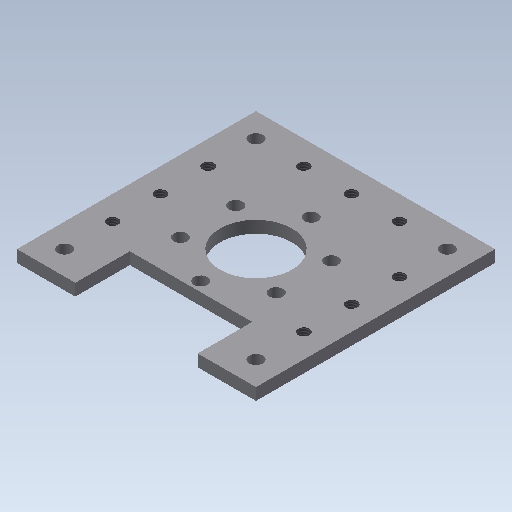
# Autodesk Inventor part: basenueva(5x5)
Saved by Autodesk Inventor 2020 (Build 240168000, 168)
## iProperties
Created: 2016-08-12
Part Number: basenueva(5x5)
Material: Genérico
Document SubType Name: Modeling
Designer: Diego Martinez
Density: 1 g/cm^3
Appearance: Por defecto
Author: Diego Martinez
Autodesk Inventor part; units mm, degrees
ref_plane "YZ Plane" through (0, 0, 0) normal (1, 0, 0) x (0, 1, 0)
ref_plane "XZ Plane" through (0, 0, 0) normal (0, 1, 0) x (-1, 0, 0)
ref_plane "XY Plane" through (0, 0, 0) normal (0, 0, 1) x (1, 0, 0)
sketch "Sketch3" plane through (0, 0, 0) normal (0, 1, 0) x (-1, 0, 0)
  circle A0 centre (0, 29.3624) radius 3.6195
  circle A1 centre (0, 29.3624) radius 3.6195
  circle A2 centre (25.4286, 14.6812) radius 3.6195
  circle A3 centre (-25.4286, 14.6812) radius 3.6195
  circle A4 centre (-25.4286, -14.6812) radius 3.6195
  circle A5 centre (0, -29.3624) radius 3.6195
  circle A6 centre (25.4286, -14.6812) radius 3.6195
  circle A7 centre (-25.4286, 14.6812) radius 3.6195
  circle A8 centre (-25.4286, -14.6812) radius 3.6195
  circle A9 centre (0, -29.3624) radius 3.6195
  circle A10 centre (25.4286, -14.6812) radius 3.6195
  circle A11 centre (25.4286, 14.6812) radius 3.6195
  line L0 (-63.5, 63.5) -> (63.5, 63.5)
  line L1 (63.5, 63.5) -> (63.5, -63.5)
  line L2 (63.5, -63.5) -> (-63.5, -63.5)
  line L3 (-63.5, -63.5) -> (-63.5, 63.5)
  line L4 (-63.5, 63.5) -> (63.5, -63.5) construction
  line L5 (63.5, 63.5) -> (-63.5, -63.5) construction
  point P0 (0, 0)
  dimension "d104" = 127
  dimension "d105" = 127
  constraints: 12 centre point, 12 end point, 6 coincident, 6 concentric, 2 midpoint, 2 parallel, 1 horizontal, 1 perpendicular
  measures "d104" distance of L1.end L2.end
  measures "d105" distance of L0.end L1.end
extrude "Extrusion1" add sketch "Sketch3" along normal blind 6.35
sketch "Sketch4" plane through (0, 0, 0) normal (0, -1, 0) x (1, 0, 0)
  circle A0 centre (-50.8, -50.8) radius 3
  line L0 (-63.5, -63.5) -> (-63.5, 63.5) projected
  line L1 (63.5, -63.5) -> (-63.5, -63.5) projected
  circle A1 centre (50.8, -50.8) radius 3
  line L2 (63.5, 63.5) -> (63.5, -63.5) projected
  circle A2 centre (50.8, 50.8) radius 3
  line L3 (-63.5, 63.5) -> (63.5, 63.5) projected
  circle A3 centre (-50.8, 50.8) radius 3
  point P0 (0, 0)
  dimension "d106" = 6
  dimension "d107" = 12.7
  dimension "d108" = 12.7
  dimension "d109" = 6
  dimension "d110" = 12.7
  dimension "d111" = 12.7
  dimension "d112" = 6
  dimension "d113" = 12.7
  dimension "d114" = 12.7
  dimension "d115" = 6
  dimension "d116" = 12.7
  dimension "d117" = 12.7
  constraints: 4 centre point
  measures "d106" diameter of A0
  measures "d107" distance from line of L0 A0.centre
  measures "d108" distance from line of A0.centre L1
  measures "d109" diameter of A1
  measures "d110" distance from line of L2 A1.centre
  measures "d111" distance from line of L1 A1.centre
  measures "d112" diameter of A2
  measures "d113" distance from line of L3 A2.centre
  measures "d114" distance from line of L2 A2.centre
  measures "d115" diameter of A3
  measures "d116" distance from line of L3 A3.centre
  measures "d117" distance from line of A3.centre L0
hole "Hole6" at (-50.8, 0, 50.8) direction (0, 1, 0) diameter 6 end through all
hole "Hole7" at (50.8, 0, 50.8) direction (0, 1, 0) diameter 6 end through all
hole "Hole8" at (50.8, 0, -50.8) direction (0, 1, 0) diameter 6 end through all
hole "Hole9" at (-50.8, 0, -50.8) direction (0, 1, 0) diameter 6 end through all
hole "Hole10" at (0, 0, 0) direction (0, 1, 0) diameter 38.1 end through all
pattern_linear "Rectangular Pattern5" count 4 spacing 25.4 along (0, 0, -1) of "Hole6"
pattern_linear "Rectangular Pattern6" count 4 spacing 25.4 along (1, 0, 0) of "Hole6"
pattern_linear "Rectangular Pattern7" count 4 spacing 25.4 along (0, 0, -1) of "Hole7"
pattern_linear "Rectangular Pattern8" count 4 spacing 25.4 along (-1, 0, 0) of "Hole8"
thread "Thread21" size "1/4-20 UNC" class "2B" standard "ANSI Unified Screw Threads" full length
thread "Thread22" size "1/4-20 UNC" class "2B" standard "ANSI Unified Screw Threads" full length
thread "Thread23" size "1/4-20 UNC" class "2B" standard "ANSI Unified Screw Threads" full length
thread "Thread24" size "1/4-20 UNC" class "2B" standard "ANSI Unified Screw Threads" full length
thread "Thread25" size "1/4-20 UNC" class "2B" standard "ANSI Unified Screw Threads" full length
thread "Thread26" size "1/4-20 UNC" class "2B" standard "ANSI Unified Screw Threads" full length
thread "Thread27" size "1/4-20 UNC" class "2B" standard "ANSI Unified Screw Threads" full length
thread "Thread28" size "1/4-20 UNC" class "2B" standard "ANSI Unified Screw Threads" full length
thread "Thread29" size "1/4-20 UNC" class "2B" standard "ANSI Unified Screw Threads" full length
thread "Thread30" size "1/4-20 UNC" class "2B" standard "ANSI Unified Screw Threads" full length
thread "Thread31" size "1/4-20 UNC" class "2B" standard "ANSI Unified Screw Threads" full length
thread "Thread32" size "1/4-20 UNC" class "2B" standard "ANSI Unified Screw Threads" full length
sketch "Sketch6" plane through (0, 6.35, 0) normal (0, 1, 0) x (1, 0, 0)
  line L0 (-32.5, -92.5) -> (32.5, -92.5)
  line L1 (32.5, -92.5) -> (32.5, -34.5)
  line L2 (32.5, -34.5) -> (-32.5, -34.5)
  line L3 (-32.5, -34.5) -> (-32.5, -92.5)
  line L4 (-63.5, -63.5) -> (63.5, -63.5) projected
  line L5 (-32.5, -92.5) -> (32.5, -34.5) construction
  line L6 (32.5, -92.5) -> (-32.5, -34.5) construction
  point P0 (0, 0)
  point P1 (0, -63.5)
  dimension "d189" = 65
  dimension "d232" = 58
  constraints: 12 end point, 3 midpoint, 2 parallel, 1 horizontal, 1 perpendicular
  measures "d189" distance of L2.end L1.end
  measures "d232" distance of L0.end L1.end
extrude "Extrusion2" cut sketch "Sketch6" against normal blind 25.4
sketch "Sketch7" plane through (0, 6.35, 0) normal (0, 1, 0) x (1, 0, 0)
  circle A0 centre (-50.8, -50.8) radius 3
  line L0 (-63.5, -63.5) -> (-63.5, 63.5)
  line L1 (63.5, -63.5) -> (-63.5, -63.5)
  circle A1 centre (50.8, -50.8) radius 3
  line L2 (63.5, 63.5) -> (63.5, -63.5)
  circle A2 centre (50.8, 50.8) radius 3
  line L3 (-63.5, 63.5) -> (63.5, 63.5)
  circle A3 centre (-50.8, 50.8) radius 3
  point P0 (0, 0)
  point P1 (0, 0)
  dimension "d192" = 6
  dimension "d193" = 12.7
  dimension "d194" = 12.7
  dimension "d195" = 6
  dimension "d196" = 12.7
  dimension "d197" = 12.7
  dimension "d198" = 6
  dimension "d199" = 12.7
  dimension "d200" = 12.7
  dimension "d201" = 6
  dimension "d202" = 12.7
  dimension "d203" = 12.7
  constraints: 8 end point, 4 centre point
  measures "d192" diameter of A0
  measures "d193" distance from line of L0 A0.centre
  measures "d194" distance from line of A0.centre L1
  measures "d195" diameter of A1
  measures "d196" distance from line of L2 A1.centre
  measures "d197" distance from line of L1 A1.centre
  measures "d198" diameter of A2
  measures "d199" distance from line of L3 A2.centre
  measures "d200" distance from line of L2 A2.centre
  measures "d201" diameter of A3
  measures "d202" distance from line of L3 A3.centre
  measures "d203" distance from line of A3.centre L0
hole "Hole11" at (-50.8, 6.35, -50.8) direction (0, -1, 0) diameter 7.3 end through all
hole "Hole12" at (50.8, 6.35, -50.8) direction (0, -1, 0) diameter 7.3 end through all
hole "Hole13" at (50.8, 6.35, 50.8) direction (0, -1, 0) diameter 7.3 end through all
hole "Hole14" at (-50.8, 6.35, 50.8) direction (0, -1, 0) diameter 7.3 end through all
body "Solid1"
